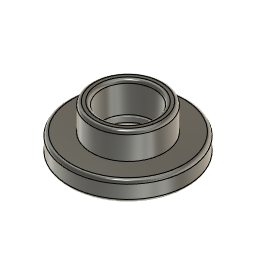
WasherForHololens (Autodesk Fusion 360 design; units mm, degrees)
Autodesk Fusion 360 part; units mm, degrees
sketch "Sketch1" plane through (0, 0, 0) normal (0, 0, 1) x (1, 0, 0)
  circle A0 centre (0, 0) radius 4.5
  dimension "d1" = 9
  constraint coincident A0.centre origin
  measures "d1" diameter of A0
extrude "Extrude1" add sketch "Sketch1" along normal blind 1.5
sketch "Sketch2" plane through (0, 0, 1.5) normal (0, 0, 1) x (-1, 0, 0)
  circle A0 centre (0, 0) radius 4.5
  circle A1 centre (0, 0) radius 2.75
  circle A2 centre (0, 0) radius 4.5
  circle A3 centre (0, 0) radius 1.875
  circle A4 centre (0, 0) radius 4.5
  dimension "d4" = 5.5
  constraint coincident A0.centre A1.centre
  measures "d4" diameter of A1
extrude "Extrude2" add sketch "Sketch2" along normal blind 2 contours A1 | A3
sketch "Sketch3" plane through (0, 0, 0) normal (0, 0, -1) x (1, 0, 0)
  circle A0 centre (0, 0) radius 4.5
  circle A1 centre (0, 0) radius 1.875
  dimension "d7" = 3.75
  constraint coincident A0.centre A1.centre
  measures "d7" diameter of A1
extrude "Extrude3" cut sketch "Sketch3" against normal blind 4 draft 2.4 contours A1
sketch "Sketch4" plane through (0, 0, 0) normal (0, 0, -1) x (1, 0, 0)
  circle A0 centre (0, 0) radius 1.875
  circle A1 centre (0, 0) radius 4.5
  circle A2 centre (0, 0) radius 2.625
  dimension "d10" = 5.25
  constraint coincident A0.centre A1.centre
  measures "d10" diameter of A2
extrude "Extrude4" cut sketch "Sketch4" against normal blind 1 contours A2
fillet "Fillet1" radius 0.25 1 edges at (-1.7872, 0.6932, 1)
fillet "Fillet2" radius 0.25 1 edges at (-2.4474, -0.9492, 0)
fillet "Fillet3" radius 0.25 4 edges at (-4.1955, -1.6273, 1.5) (-4.1955, -1.6273, 0) (2.5639, 0.9944, 3.5) (-1.8849, 0.7311, 3.5)
